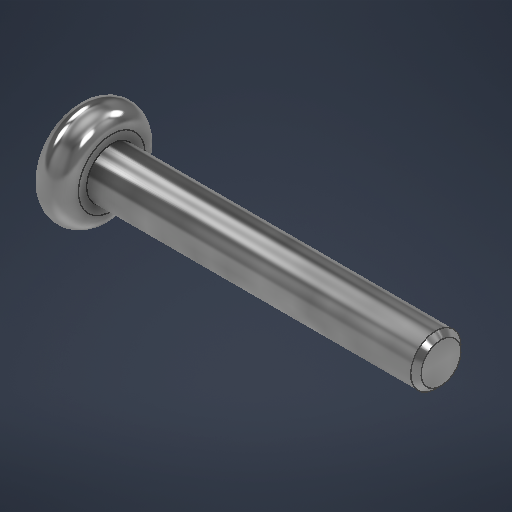
# Autodesk Inventor part: Винт М3х19
Saved by Autodesk Inventor 2025 (Build 290162010, 162A)
## iProperties
Created: 2025-01-11
Part Number: Винт М3х19
Material: Типовые
Document SubType Name: Modeling
Designer: Edward_Higgins
Density: 1 g/cm^3
Appearance: По умолчанию
Author: Edward_Higgins
Autodesk Inventor part; units mm, degrees
ref_plane "YZ Plane" through (0, 0, 0) normal (1, 0, 0) x (0, 1, 0)
ref_plane "XZ Plane" through (0, 0, 0) normal (0, 1, 0) x (-1, 0, 0)
sketch "Эскиз1" plane through (0, 0, 0) normal (0, 0, 1) x (1, 0, 0)
  line L0 (0, 0) -> (-21.3726, 0)
  arc A0 (-19, 1.9227) -> (-21, 2.2534) centre (-20.0273, 1.9227) ccw
  line L1 (-19, 1.9227) -> (-19, 1.45)
  line L2 (-19, 1.45) -> (0, 1.45)
  line L3 (0, 1.45) -> (0, 0)
  line L4 (-21.6724, 2.95) -> (-19.1128, 2.95)
  arc A1 (-21, 2.2534) -> (-21.3726, 0) centre (-14.3726, 0) ccw
  dimension "d0" = 2.9
  dimension "d1" = 5.9
  dimension "d2" = 2
  dimension "d3" = 19
  dimension "d4" = 7
  constraints: 10 end point, 4 point on circle, 3 tangent, 2 centre point, 2 horizontal, 2 perpendicular, 1 line through centre
  measures "d0" diameter of L2 L0
  measures "d1" diameter of L4 L0
  measures "d2" distance from line of A0.end L1
  measures "d3" distance between parallel lines of L3 L1
  measures "d4" radius of A1
revolve "Вращение1" add sketch "Эскиз1" angle 360 about axis through (0, 0, 0) along (-1, 0, 0)
chamfer "Фаска1" distance 0.3 angle 45 1 edges at (0, -1.45, 0)
ref_plane "РабПлоскость2" through (-21.3726, 0, 0) normal (1, 0, 0) x (0, 0, -1)
sketch "Эскиз2" plane through (-21.3726, 0, 0) normal (1, 0, 0) x (0, 0, -1)
  line L0 (-0.4, 1.5) -> (0.4, 1.5)
  line L1 (0.4, 1.5) -> (0.4, -1.5)
  line L2 (0.4, -1.5) -> (-0.4, -1.5)
  line L3 (-0.4, -1.5) -> (-0.4, 1.5)
  line L4 (-1.5, 0.4) -> (1.5, 0.4)
  line L5 (1.5, 0.4) -> (1.5, -0.4)
  line L6 (1.5, -0.4) -> (-1.5, -0.4)
  line L7 (-1.5, -0.4) -> (-1.5, 0.4)
  point P0 (0, 0)
  point P1 (0, 1.5)
  point P2 (0, 0.4)
  point P3 (-1.5, 0)
  point P4 (-0.4, 0)
  point P5 (0.4, 0.4)
  point P6 (-0.4, 0.4)
  point P7 (-0.4, -0.4)
  point P8 (0.4, -0.4)
  dimension "d10" = 0.8
  dimension "d11" = 3
  constraints: 16 end point, 4 midpoint, 4 parallel, 4 perpendicular, 2 horizontal, 2 horizontal alignment, 2 vertical alignment
  measures "d10" distance of L6.end L4.start
  measures "d11" distance of L4.start L4.end
extrude "Выдавливание1" cut sketch "Эскиз2" along normal blind 1.2
